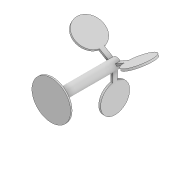
# Autodesk Inventor part: manometro idealmente
Saved by Autodesk Inventor 2022 (Build 260153000, 153)
## iProperties
Created: 2025-08-06
Part Number: manometro idealmente
Material: Generic
Document SubType Name: Modeling
Designer: sacchie
Density: 1 g/cm^3
Appearance: Default
Author: sacchie
Autodesk Inventor part; units mm, degrees
ref_plane "YZ Plane" through (0, 0, 0) normal (1, 0, 0) x (0, 1, 0)
ref_plane "XZ Plane" through (0, 0, 0) normal (0, 1, 0) x (-1, 0, 0)
ref_plane "XY Plane" through (0, 0, 0) normal (0, 0, 1) x (1, 0, 0)
sketch "Sketch1" plane through (0, 0, 0) normal (0, 0, 1) x (1, 0, 0)
  circle A0 centre (0, 0) radius 40
  dimension "d0" = 80
  constraints: 1 centre point, 1 coincident
  measures "d0" diameter of A0
extrude "Extrusion1" add sketch "Sketch1" along normal blind 3
sketch "Sketch2" plane through (0, 0, 3) normal (0, 0, 1) x (1, 0, 0)
  circle A0 centre (0, 0) radius 10
  dimension "d3" = 20
  constraints: 1 centre point, 1 coincident
  measures "d3" diameter of A0
extrude "Extrusion2" add sketch "Sketch2" against normal blind 160
sketch "Sketch3" plane through (0, 0, 0) normal (1, 0, 0) x (0, 1, 0)
  circle A0 centre (-59.9652, -126.9652) radius 30.0348
  line L0 (-10, -157) -> (10, -157) projected
  line L1 (0, -157) -> (0, -174.595) construction
  line L2 (-90, -126.9652) -> (-90, -88.517)
  line L3 (-59.9652, -126.9652) -> (0, -126.9652) construction
  line L4 (0, -126.9652) -> (0, -131.9652)
  line L5 (0, -131.9652) -> (-30.3494, -131.9652)
  line L6 (0, -126.9652) -> (0, -121.9652)
  line L7 (0, -121.9652) -> (-30.3494, -121.9652)
  point P0 (0, 0)
  dimension "d8" = 90
  dimension "d9" = 5
  dimension "d10" = 5
  constraints: 14 end point, 3 perpendicular, 3 point on circle, 3 vertical, 1 centre point, 1 horizontal, 1 midpoint, 1 tangent
  measures "d8" distance between parallel lines of L1 L2
  measures "d9" distance of L3.end L4.end
  measures "d10" distance of L3.end L6.end
extrude "Extrusion3" add sketch "Sketch3" along normal mid plane 4
sketch "Sketch4" plane through (0, 0, -157) normal (0, 0, -1) x (-1, 0, 0)
  circle A0 centre (-13.7706, 13.7706) radius 35.6894
  point P0 (0, 0)
  constraints: 1 centre point
extrude "Extrusion4" cut sketch "Sketch4" against normal up to surface (25.0348 mm away)
pattern_circular "Circular Pattern1" count 3 over 360 about axis through (0, 0, 3) along (0, 0, -1) of "Extrusion3"
body "Solid1"
